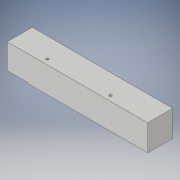
# Autodesk Inventor part: StandoffBlocks
Saved by Autodesk Inventor 2019 (Build 230136000, 136)
## iProperties
Created: 2019-09-28
Part Number: StandoffBlocks
Material: Generic
Document SubType Name: Modeling
Designer: james
Density: 1 g/cm^3
Appearance: Default
Author: james
Autodesk Inventor part; units mm, degrees
ref_plane "YZ Plane" through (0, 0, 0) normal (1, 0, 0) x (0, 1, 0)
ref_plane "XZ Plane" through (0, 0, 0) normal (0, 1, 0) x (-1, 0, 0)
ref_plane "XY Plane" through (0, 0, 0) normal (0, 0, 1) x (1, 0, 0)
sketch "Sketch1" plane through (0, 0, 0) normal (1, 0, 0) x (0, 1, 0)
  line L0 (0, 0) -> (32.8422, 0)
  line L1 (32.8422, 0) -> (32.8422, 31.75)
  line L2 (32.8422, 31.75) -> (0, 31.75)
  line L3 (0, 31.75) -> (0, 0)
  dimension "d0" = 32.8422
  dimension "d1" = 31.75
  constraints: 8 end point, 2 parallel, 1 horizontal, 1 perpendicular
  measures "d0" distance of L1.end L2.end
  measures "d1" distance of L0.end L1.end
extrude "Extrusion1" add sketch "Sketch1" along normal blind 127
sketch "Sketch2" plane through (0, 32.8422, 31.75) normal (0, 1, 0) x (1, 0, 0)
  line L0 (0, 0) -> (127, 0) projected
  line L1 (0, 31.75) -> (0, 0) projected
  point P0 (19.05, 6.35)
  point P1 (99.05, 6.35)
  dimension "d4" = 0
  dimension "d5" = 6.35
  dimension "d6" = 80
  dimension "d7" = 19.05
  measures "d4" vertical distance of point (99.05, 6.35) point (19.05, 6.35)
  measures "d5" distance from line of L0 point (99.05, 6.35)
  measures "d6" distance of point (99.05, 6.35) point (19.05, 6.35)
  measures "d7" distance from line of L1 point (19.05, 6.35)
hole "Hole1" at (19.05, 32.8422, 25.4) at (99.05, 32.8422, 25.4) direction (0, -1, 0) diameter 3.175 end through all
sketch "Sketch3" plane through (127, 0, 0) normal (1, 0, 0) x (0, 0, -1)
  line L0 (-31.75, 32.8422) -> (0, 32.8422)
  line L1 (0, 32.8422) -> (0, 0)
  line L2 (0, 0) -> (-31.75, 0)
  line L3 (-31.75, 0) -> (-31.75, 32.8422)
  line L4 (0, 32.8422) -> (-31.75, 32.8422) projected
  line L5 (-31.75, 32.8422) -> (-31.75, 0) projected
  dimension "d15" = 0
  dimension "d16" = 0
  constraints: 8 end point, 2 parallel, 1 horizontal, 1 perpendicular
  measures "d15" distance between parallel lines of L4 L0
  measures "d16" distance between parallel lines of L5 L3
extrude "Extrusion2" add sketch "Sketch3" along normal blind 25.4
sketch "Sketch4" plane through (0, 0, 0) normal (-1, 0, 0) x (0, 0, 1)
  line L0 (0, 32.8422) -> (31.75, 32.8422) projected
  line L1 (0, 32.8422) -> (31.75, 32.8422)
  line L2 (31.75, 32.8422) -> (31.75, 1.0922)
  line L3 (31.75, 1.0922) -> (0, 1.0922)
  line L4 (0, 1.0922) -> (0, 32.8422)
  point P0 (0, 0)
  constraints: 8 end point, 2 parallel, 1 horizontal, 1 perpendicular
extrude "Extrusion3" add sketch "Sketch4" along normal blind 25.4
body "Solid1"
